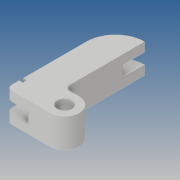
# Autodesk Inventor part: viseur_reglable_piece
Saved by Autodesk Inventor 2019 (Build 230136000, 136)
## iProperties
Created: 2019-01-06
Part Number: viseur_reglable_piece
Material: Générique
Document SubType Name: Modeling
Designer: Theo
Density: 1 g/cm^3
Appearance: Par défaut
Author: Theo
Autodesk Inventor part; units mm, degrees
ref_plane "YZ Plane" through (0, 0, 0) normal (1, 0, 0) x (0, 1, 0)
ref_plane "XZ Plane" through (0, 0, 0) normal (0, 1, 0) x (-1, 0, 0)
ref_plane "XY Plane" through (0, 0, 0) normal (0, 0, 1) x (1, 0, 0)
sketch "Esquisse3" plane through (0, 0, 0) normal (0, 1, 0) x (-1, 0, 0)
  line L0 (4, 0) -> (-4, 0)
  line L1 (-4, 0) -> (-4, -30)
  arc A0 (-4, -30) -> (4, -22) centre (-4, -22) ccw
  line L2 (4, 0) -> (4, -22)
  point P0 (0, 0)
  point P1 (0, 0)
  dimension "d21" = 8
  dimension "d22" = 30
  constraints: 6 end point, 2 point on circle, 2 vertical, 1 centre point, 1 coincident, 1 horizontal, 1 midpoint, 1 point on line, 1 tangent
  measures "d21" distance of L0.start L0.end
  measures "d22" distance of L0.end L1.end
extrude "Extrusion2" add sketch "Esquisse3" along normal mid plane 8
sketch "Esquisse4" plane through (0, 0, 0) normal (0, 1, 0) x (-1, 0, 0)
  line L0 (-4, 0) -> (4, 0) projected
  line L1 (4, 0) -> (4, -22) projected
  arc A0 (-4, -30) -> (4, -22) centre (-4, -22) ccw projected
  line L2 (-4, -30) -> (-4, 0) projected
  line L3 (-4, -30) -> (-4, 0) projected
  line L4 (-2, -22) -> (-2, 0)
  arc A1 (-4, -24) -> (-2, -22) centre (-4, -22) ccw
  point P0 (0, 0)
  dimension "d26" = 6
  dimension "d27" = 6
  constraints: 2 end point, 2 point on circle, 2 point on line, 1 centre point, 1 horizontal alignment, 1 tangent, 1 vertical
  measures "d26" distance between parallel lines of L1 L4
  measures "d27" distance of L2.start A1.start
extrude "Extrusion3" cut sketch "Esquisse4" along normal mid plane 3 contours L0 L1 A0 L2 A1 L4
sketch "Esquisse5" plane through (0, 4, 0) normal (0, 1, 0) x (1, 0, 0)
  line L0 (4, 30) -> (4, 0) projected
  line L1 (4, 0) -> (12, 0)
  line L2 (12, 0) -> (12, 8)
  line L3 (12, 8) -> (4, 8)
  line L4 (4, 8) -> (4, 0)
  point P0 (0, 0)
  dimension "d30" = 8
  dimension "d31" = 8
  constraints: 8 end point, 2 parallel, 1 horizontal, 1 perpendicular
  measures "d30" distance of L2.end L3.end
  measures "d31" distance of L1.end L2.end
extrude "Extrusion4" add sketch "Esquisse5" against normal up to surface (8 mm away)
sketch "Esquisse6" plane through (0, 4, 0) normal (0, 1, 0) x (1, 0, 0)
  line L0 (-4, 0) -> (12, 0) projected
  line L1 (12, 0) -> (12, 8) projected
  line L2 (4, 8) -> (4, 30) projected
  point P0 (0, 0)
  point P1 (8, 4)
  dimension "d34" = 4
  dimension "d47" = 4
  measures "d34" distance from line of L0 point (8, 4)
  measures "d47" distance from line of point (8, 4) L2
hole "Perçage2" at (8, 4, -4) direction (0, -1, 0) diameter 4 depth 8
fillet "Congé2" radius 1.5 3 edges at (-4, 2.75, 0) (-4, -2.75, 0) (4, 0, -8)
fillet "Congé3" radius 4 2 edges at (12, 0, 0) (12, 0, -8)
sketch "Esquisse7" plane through (-4, 1.5, -22) normal (-1, 0, 0) x (0, 0, 1)
  line L0 (16, 2.5) -> (20, 2.5) projected
  line L1 (20.5, -5.5) -> (0, -5.5) projected
  line L2 (20.5, -3) -> (0, -3) projected
  line L3 (17.5, -5.5) -> (18.5, -5.5)
  line L4 (18.5, -5.5) -> (18.5, -3)
  line L5 (18.5, -3) -> (17.5, -3)
  line L6 (17.5, -3) -> (17.5, -5.5)
  line L7 (0, 0) -> (20.5, 0) projected
  line L8 (0, 2.5) -> (20.5, 2.5) projected
  line L9 (17.5, 0) -> (18.5, 0)
  line L10 (18.5, 0) -> (18.5, 2.5)
  line L11 (18.5, 2.5) -> (17.5, 2.5)
  line L12 (17.5, 2.5) -> (17.5, 0)
  line L13 (20, -5.5) -> (16, -5.5) projected
  line L14 (16, 2.5) -> (20, 2.5) projected
  point P0 (22, -1.5)
  point P1 (18, 2.5)
  dimension "d49" = 1
  constraints: 16 end point, 6 point on line, 4 parallel, 2 horizontal, 2 midpoint, 2 perpendicular
  measures "d49" distance between parallel lines of L10 L12
extrude "Extrusion5" cut sketch "Esquisse7" against normal blind 1
